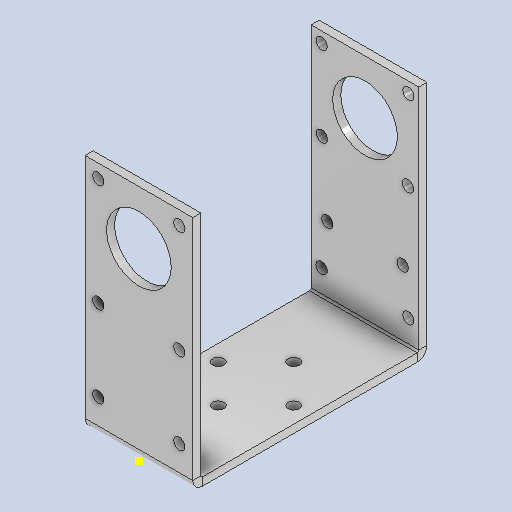
# Autodesk Inventor part: axis_19_top_frame
Saved by Autodesk Inventor 2025.2 (Build 292293000, 293)
## iProperties
Created: 2025-05-06
Part Number: axis_19_top_frame
Material: Aluminum 6061-AHC
Document SubType Name: Sheet Metal
Designer: LG
Density: 2.7 g/cm^3
Sheet Metal Rule: Default_mm
Appearance: Aluminum - Dark
Author: LG
Autodesk Inventor part; units mm, degrees
ref_plane "YZ Plane" through (0, 0, 0) normal (1, 0, 0) x (0, 1, 0)
ref_plane "XZ Plane" through (0, 0, 0) normal (0, 1, 0) x (-1, 0, 0)
ref_plane "XY Plane" through (0, 0, 0) normal (0, 0, 1) x (1, 0, 0)
sketch "Sketch1" plane through (0, 0, 0) normal (0, 1, 0) x (-1, 0, 0)
  line L0 (-10, 20.25) -> (10, 20.25)
  line L1 (10, 20.25) -> (10, -20.25)
  line L2 (10, -20.25) -> (-10, -20.25)
  line L3 (-10, -20.25) -> (-10, 20.25)
  line L4 (-10, 20.25) -> (10, -20.25) construction
  line L5 (10, 20.25) -> (-10, -20.25) construction
  point P0 (0, 0)
  dimension "d0" = 40.5
  dimension "d1" = 20
  measures "d0" distance of L0.end L1.end
  measures "d1" distance of L1.end L2.end
extrude "Plate1" add sketch "Sketch1" along normal blind 1.5
sketch "Sketch2" plane through (-10, 0, -21.75) normal (0, 0, 1) x (1, 0, 0)
  line L0 (20, 0) -> (0, 0)
  line L1 (0, 0) -> (0, 44.1)
  line L2 (0, 44.1) -> (20, 44.1)
  line L3 (20, 44.1) -> (20, 0)
  constraints: 8 end point
edge flange "Flange1" height 44.1 angle 90 thickness 1.5 bend radius 0.31 thickness toward (0, 0, 1) relief straight relief width 1.5 relief depth 0.75 corner gap 0.31 corner form 0 edges at (0, 1.5, -20.25) (0, 1.5, 20.25) wall of the first edge with corners at (10, 0, -21.75) (-10, 0, -21.75) (-10, 44.1, -21.75) (10, 44.1, -21.75)
bend "Bend1"
corner "Corner1"
sketch "Sketch3" plane through (0, 1.5, 0) normal (0, 1, 0) x (1, 0, 0)
  circle A0 centre (7, 0) radius 0.7835 projected
  circle A1 centre (0, -7) radius 0.7835 projected
  circle A2 centre (-7, 0) radius 0.7835 projected
  circle A3 centre (0, 7) radius 0.7835 projected
  point P0 (0, 0)
hole "Hole1" at (0, 1.5, 7) at (7, 1.5, 0) at (-7, 1.5, 0) at (0, 1.5, -7) direction (0, -1, 0) diameter 2.1 depth 1.5
sketch "Sketch4" plane through (-10, 44.1, -20.25) normal (0, 0, 1) x (1, 0, 0)
  point P0 (10, -44.1)
sketch "Sketch5" plane through (-10, 44.1, -20.25) normal (0, 0, 1) x (1, 0, 0)
  point P0 (10, -44.1)
sketch "Sketch11" plane through (-10, 44.1, 21.75) normal (0, 0, 1) x (1, 0, 0)
  point P0 (10, -44.1)
sketch "Sketch20" plane through (-10, 1.81, 21.75) normal (0, 0, 1) x (1, 0, 0)
  point P0 (10, -1.81)
sketch "Sketch21" plane through (-10, 1.81, 21.75) normal (0, 0, 1) x (1, 0, 0)
  circle A0 centre (17.525, 39.79) radius 0.7835
  circle A1 centre (17.525, 19.79) radius 0.7835
  circle A2 centre (17.525, 4.69) radius 0.7835
  circle A3 centre (2.475, 39.79) radius 0.7835
  circle A4 centre (2.475, 19.79) radius 0.7835
  circle A5 centre (2.475, 4.69) radius 0.7835
  point P0 (10, -1.81)
  constraints: 6 centre point, 12 other
hole "Hole6" at (7.525, 41.6, 21.75) at (-7.525, 41.6, 21.75) at (7.525, 21.6, 21.75) at (-7.525, 21.6, 21.75) at (7.525, 6.5, 21.75) at (-7.525, 6.5, 21.75) direction (0, 0, -1) diameter 2.1 depth 1.5
sketch "Sketch22" plane through (10, 1.81, -21.75) normal (0, 0, -1) x (-1, 0, 0)
  circle A0 centre (1.93, 4.19) radius 0.7835
  circle A1 centre (3, 12.17) radius 0.7835
  circle A2 centre (2, 25.39) radius 0.7835
  circle A3 centre (18.07, 4.19) radius 0.7835
  circle A4 centre (17, 12.17) radius 0.7835
  circle A5 centre (18, 25.39) radius 0.7835
  point P0 (10, -1.81)
  constraints: 6 centre point, 12 other
hole "Hole7" at (8.07, 6, -21.75) at (7, 13.98, -21.75) at (-8.07, 6, -21.75) at (-7, 13.98, -21.75) at (8, 27.2, -21.75) at (-8, 27.2, -21.75) direction (0, 0, 1) diameter 2.1 depth 1.5
sketch "Sketch23" plane through (-10, 44.1, 21.75) normal (0, 0, 1) x (1, 0, 0)
  circle A0 centre (10, -10) radius 6
  point P0 (10, -44.1)
  constraints: 1 centre point, 2 other
extrude "Cut9" cut sketch "Sketch23" against normal blind 1.5
sketch "Sketch24" plane through (10, 44.1, -21.75) normal (0, 0, -1) x (-1, 0, 0)
  circle A0 centre (10, -10) radius 6
  point P0 (10, -44.1)
  constraints: 1 centre point, 2 other
extrude "Cut10" cut sketch "Sketch24" against normal blind 1.5
sketch "Sketch25" plane through (10, 44.1, -21.75) normal (0, 0, -1) x (-1, 0, 0)
  circle A0 centre (18.07, -2) radius 0.7835
  circle A1 centre (1.93, -2) radius 0.7835
  point P0 (10, -44.1)
  constraints: 2 centre point, 4 other
hole "Hole8" at (8.07, 42.1, -21.75) at (-8.07, 42.1, -21.75) direction (0, 0, 1) diameter 2.1 depth 1.5
equation "\"d18\" = Thickness"
equation "\"d71\" = Thickness"
equation "\"d78\" = Thickness"
equation "\"d80\" = Thickness"
equation "\"d82\" = Thickness"
equation "\"d89\" = Thickness"
equation "\"d2\" = Thickness"
equation "\"d3\" = BendReliefWidth"
equation "\"d4\" = BendReliefDepth"
equation "\"d5\" = MinimumRemnant"
equation "\"d6\" = TransitionRadius"
equation "\"d9\" = BendRadius"
equation "\"d10\" = CornerReliefSize"
equation "\"d11\" = GapSize"
equation "\"d12\" = JacobiRadiusSize"
equation "\"BendReliefWidth\" = Thickness"
equation "\"BendReliefDepth\" = 0.5 * Thickness"
equation "\"CornerReliefSize\" = 4 * Thickness"
equation "\"MinimumRemnant\" = 2 * Thickness"
equation "\"TransitionRadius\" = BendRadius"
equation "\"JacobiRadiusSize\" = BendRadius"
equation "\"GapSize\" = Thickness"
equation "\"Thickness\" = 1.5"
equation "\"BendRadius\" = 0.31"
body "Solid1"
